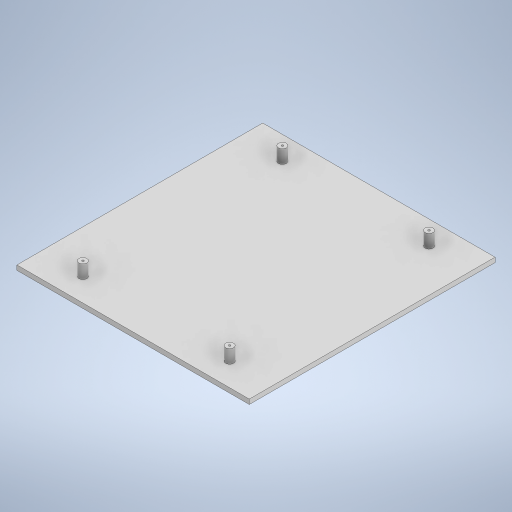
# Autodesk Inventor part: Cabinet - back
Saved by Autodesk Inventor 2024.3 (Build 283343000, 343)
## iProperties
Created: 2025-03-25
Part Number: Cabinet - back
Material: Všeobecné
Document SubType Name: Modeling
Designer: admin
Density: 1 g/cm^3
Appearance: Výchozí
Author: admin
Autodesk Inventor part; units mm, degrees
sketch "Náčrt1" plane through (0, 0, 0) normal (0, 1, 0) x (-1, 0, 0)
  line L0 (86.5, 91.5) -> (-86.5, 91.5)
  line L1 (-86.5, 91.5) -> (-86.5, -91.5)
  line L2 (-86.5, -91.5) -> (86.5, -91.5)
  line L3 (86.5, -91.5) -> (86.5, 91.5)
  line L4 (121.1, 0) -> (-121.1, 0) projected
  line L5 (0, -128.1) -> (0, 128.1) projected
  point P0 (0, 0)
  dimension "d0" = 183
  dimension "d1" = 173
  constraints: 8 end point, 2 parallel, 1 horizontal, 1 perpendicular, 2 other
  measures "d0" distance of L2.end L0.start
  measures "d1" distance of L0.start L0.end
extrude "Vysunutí1" add sketch "Náčrt1" along normal blind 3.5
sketch "Náčrt2" plane through (0, 3.5, 0) normal (0, 1, 0) x (1, 0, 0)
  circle A0 centre (-54.61, -74.259) radius 3
  line L0 (0, 128.1) -> (0, -128.1) projected
  line L1 (-121.1, 0) -> (121.1, 0) projected
  point P0 (0, 0)
  dimension "d4" = 6
  dimension "d14" = 54.61
  dimension "d15" = 74.259
  constraints: 1 centre point
  measures "d4" diameter of A0
  measures "d14" distance from line of L0 A0.centre
  measures "d15" distance from line of L1 A0.centre
extrude "Vysunutí2" add sketch "Náčrt2" along normal blind 10
ref_plane "Pracovní rovina1" through (0, 0, 91.5) normal (1, 0, 0) x (0, 0, -1)
ref_plane "Pracovní rovina2" through (-86.5, 0, 0) normal (0, 0, 1) x (1, 0, 0)
sketch "Náčrt3" plane through (-54.61, 13.5, 74.259) normal (0, 1, 0) x (1, 0, 0)
  point P0 (54.61, 74.259)
  point P1 (0, 0)
  point P2 (0, 0)
  constraints: 1 coincident
hole "Díra1" at (-54.61, 13.5, 74.259) direction (0, -1, 0) diameter 1.5 depth 8 tip angle 118
pattern_circular "Kruhové pole1" count 2 over 360 about axis through (0, -10, 0) along (0, 1, 0) of "Vysunutí2", "Díra1"
mirror "Zrcadlit1" about plane through (0, 0, 0) normal (0, 0, 1) of "Vysunutí2", "Díra1", "Kruhové pole1"
ref_plane "Pracovní rovina5" through (0, 1.75, 0) normal (0, 1, 0) x (1, 0, 0)
ref_plane "Pracovní rovina3" through (0, 0, 0) normal (0, 0, 1) x (1, 0, 0)
